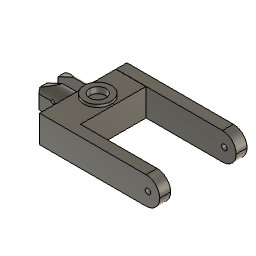
main_gear_wheel_holder (Autodesk Fusion 360 design; units mm, degrees)
Autodesk Fusion 360 part; units mm, degrees
sketch "Sketch3" plane through (0, 0, 0) normal (1, 0, 0) x (0, 1, 0)
  line L0 (-12.0524, 0) -> (11.9476, 0)
  line L1 (11.9476, 0) -> (11.9476, 8.75)
  line L2 (11.9476, 8.75) -> (-12.0524, 8.75)
  line L3 (-12.0524, 8.75) -> (-12.0524, 0)
  dimension "d7" = 8.75
  dimension "d11" = 24
  constraint horizontal L0
  constraint vertical L1
  constraint horizontal L2
  constraint vertical L3
  measures "d7" distance of L0.start L2.end
  measures "d11" distance of L0.start L0.end
extrude "Extrude3" add sketch "Sketch3" against normal blind 9 makes body 1
sketch "Sketch4" plane through (-9, 0, 0) normal (-1, 0, 0) x (0, -1, 0)
  line L0 (12.0524, 0) -> (12.0524, 8.75)
  line L1 (12.0524, 8.75) -> (-11.9476, 8.75)
  line L2 (-11.9476, 8.75) -> (-11.9476, 0)
  line L3 (-11.9476, 0) -> (12.0524, 0)
  dimension "d10" = 24
  measures "d10" distance of L0.start L2.end
sketch "Sketch5" plane through (0, 0, 0) normal (1, 0, 0) x (0, 1, 0)
  line L0 (12, 0) -> (16, 0)
  line L1 (16, 0) -> (16, 10)
  line L2 (16, 10) -> (12, 10)
  line L3 (12, 10) -> (12, 0)
  line L4 (-12, 0) -> (-16, 0)
  line L5 (-16, 0) -> (-16, 10)
  line L6 (-16, 10) -> (-12, 10)
  line L7 (-12, 10) -> (-12, 0)
  constraint horizontal L0
  constraint vertical L1
  constraint horizontal L2
  constraint vertical L3
  constraint horizontal L4
  constraint vertical L5
  constraint horizontal L6
  constraint vertical L7
extrude "Extrude4" add sketch "Sketch5" along normal blind 33 and the other way blind 9 bodies 1 makes body 2 at (5, 12, 6.6667)
extrude "Extrude5" add sketch "Sketch4" 2 faces at (-9, 13.3333, 6.6667) (-9, -5.3508, 2.9167) along normal blind 2 on bodies 1 2 bodies 2 1
sketch "Sketch6" plane through (0, 0, 8.75) normal (0, 0, 1) x (-1, 0, 0)
  line L0 (11, 12) -> (0, 12)
  line L1 (0, 12) -> (0, -11.9476)
  line L2 (0, -11.9476) -> (11, -11.9476)
  line L3 (11, -11.9476) -> (11, 12)
  circle A0 centre (5.6836, 0.0262) radius 5.0001
extrude "Extrude6" add sketch "Sketch6" along normal blind 2.25 contours A0 bodies 1
extrude "Extrude7" add 1 faces at (-5.4366, 9.6184, 8.75) along direction (0, 0, 1) blind 1.25 on bodies 1 bodies 1
sketch "Sketch7" plane through (-11, 0, 0) normal (-1, 0, 0) x (0, -1, 0)
  line L0 (-11.9476, 0) -> (16, 0)
  line L1 (16, 0) -> (16, 10)
  line L2 (16, 10) -> (-11.9476, 10)
  line L3 (-11.9476, 10) -> (-11.9476, 0)
  circle A0 centre (0, 5) radius 5
  dimension "d51" = 10
  measures "d51" diameter of A0
extrude "Extrude8" add sketch "Sketch7" along normal blind 11.25 contours A0 bodies 1
sketch "Sketch8" plane through (-22.25, 0, 0) normal (-1, 0, 0) x (0, -1, 0)
  circle A0 centre (0, 5) radius 5
  line L0 (-2, 10) -> (2, 10)
  line L1 (2, 10) -> (2, 0)
  line L2 (2, 0) -> (-2, 0)
  line L3 (-2, 0) -> (-2, 10)
  constraint horizontal L0
  constraint vertical L1
  constraint horizontal L2
  constraint vertical L3
extrude "Extrude9" cut sketch "Sketch8" against normal blind 11.25 contours A0 L1 L3 bodies 1
sketch "Sketch9" plane through (0, 0, 0) normal (0, 1, 0) x (1, 0, 0)
  circle A0 centre (-17.177, -5.0278) radius 0.6282
sketch "Sketch10" plane through (0, 0, 11) normal (0, 0, 1) x (-1, 0, 0)
  circle A0 centre (5.6836, 0.0262) radius 5.0001
  circle A1 centre (5.6836, 0.0262) radius 3
  dimension "d29" = 6
  constraint concentric A0 A1
  measures "d29" diameter of A1
extrude "Extrude11" cut sketch "Sketch10" against normal blind 2.25 contours A1 bodies 1
ref_plane "WorkPlane2" through (-22.5, 0, 0) normal (1, 0, 0) x (0, 1, 0)
sketch "Sketch11" plane through (-22.5, 0, 0) normal (1, 0, 0) x (0, 1, 0)
  line L0 (1, 10, 2) -> (6.2958, 10, 2)
  line L1 (6.2958, 10, 2) -> (6.2958, -0.0309, 2)
  line L2 (6.2958, -0.0309, 2) -> (1, -0.0309, 2)
  line L3 (1, -0.0309, 2) -> (1, 10, 2)
ref_plane "WorkPlane3" through (-20.5, 3.6479, 10) normal (-0.422618, 0, 0.906308) x (0, 1, 0)
sketch "Sketch12" plane through (-7.4916, 0, 16.0659) normal (-0.422618, 0, 0.906308) x (0, 1, 0)
  line L0 (6.5087, 8.2785) -> (-8.5877, 8.2785)
  line L1 (-8.5877, 8.2785) -> (-8.5877, 18.2785)
  line L2 (-8.5877, 18.2785) -> (6.5087, 18.2785)
  line L3 (6.5087, 18.2785) -> (6.5087, 8.2785)
  dimension "d41" = 10
  constraint horizontal L0
  constraint vertical L1
  constraint horizontal L2
  constraint vertical L3
  measures "d41" distance of L0.start L2.end
extrude "Extrude13" cut sketch "Sketch12" along normal blind 4 and the other way blind 1 bodies 1
extrude "Extrude14" cut sketch "Sketch12" along normal blind 3 and the other way blind 2 bodies 1
sketch "Sketch13" plane through (0, 0, 0) normal (0, 1, 0) x (1, 0, 0)
  circle A0 centre (28.7038, -5) radius 1
  dimension "d46" = 2
  measures "d46" diameter of A0
extrude "Extrude15" cut sketch "Sketch13" along normal mid plane 66 bodies 1 2
fillet "Fillet1" radius 5 4 edges at (33, -14, 10) (33, -14, 0) (33, 14, 10) (33, 14, 0) on bodies 1 2
sketch "Sketch14" plane through (-11, 0, 0) normal (-1, 0, 0) x (0, -1, 0)
  arc A0 (-2, 9.5826) -> (-2, 0.4174) centre (0, 5) ccw
  line L0 (-2, 9.5826) -> (-2, 0.4174)
  line L1 (-11.9476, 0) -> (16, 0)
  line L2 (16, 0) -> (16, 10)
  line L3 (16, 10) -> (-11.9476, 10)
  line L4 (-11.9476, 10) -> (-11.9476, 0)
  line L5 (2, 0.4174) -> (2, 9.5826)
  arc A1 (2, 0.4174) -> (2, 9.5826) centre (0, 5) ccw
  line L6 (-2, 5) -> (-5, 5)
  line L7 (-5, 5) -> (-5, 0)
  line L8 (-5, 0) -> (-2, 0)
  line L9 (-2, 0) -> (-2, 5)
  line L10 (2, 5) -> (5, 5)
  line L11 (5, 5) -> (5, 0)
  line L12 (5, 0) -> (2, 0)
  line L13 (2, 0) -> (2, 5)
  constraint horizontal L6
  constraint vertical L7
  constraint horizontal L8
  constraint vertical L9
  constraint coincident L1 L7.end
  constraint midpoint L0 L6.start
  constraint horizontal L10
  constraint vertical L11
  constraint horizontal L12
  constraint vertical L13
  constraint coincident L1 L11.end
  constraint midpoint L5 L10.start
extrude "Extrude16" add sketch "Sketch14" along normal blind 11.25 contours A0 L1 L7 L8 L9 | L1 A1 L11 L12 L13 bodies 1
extrude "Extrude17" cut sketch "Sketch9" along normal blind 8.5 and the other way blind 7.5 bodies 1
